Autodesk Fusion 360 part; units mm, degrees
(part 3 of 6)
  spline S34 degree 5 poles (141.8254, 60.2278) (141.8393, 60.255) (141.8664, 60.3097) (141.905, 60.3928) (141.9525, 60.5053) (142.0063, 60.6483) (142.0562, 60.7931) (142.1036, 60.939) (142.1498, 61.0854) (142.1951, 61.2323) (142.2394, 61.3795) (142.2825, 61.5272) (142.3239, 61.6756) (142.3633, 61.8248) (142.4009, 61.9748) (142.4366, 62.1255) (142.4708, 62.2767) (142.5037, 62.4284) (142.5355, 62.5806) (142.5662, 62.7331) (142.5959, 62.886) (142.6244, 63.0393) (142.6517, 63.193) (142.6778, 63.3471) (142.7027, 63.5017) (142.7265, 63.6566) (142.7491, 63.8119) (142.7707, 63.9676) (142.7913, 64.1236) (142.8108, 64.2798) (142.8294, 64.4364) (142.847, 64.5933) (142.8637, 64.7505) (142.8793, 64.908) (142.8939, 65.0657) (142.9076, 65.2238) (142.9204, 65.3821) (142.9322, 65.5407) (142.9431, 65.6995) (142.9532, 65.8586) (142.9623, 66.0179) (142.9705, 66.1775) (142.9779, 66.3372) (142.9844, 66.4972) (142.99, 66.6575) (142.9948, 66.8179) (142.9987, 66.9785) (143.0017, 67.1394) (143.004, 67.3004) (143.0054, 67.4617) (143.006, 67.6231) (143.0057, 67.7847) (143.0047, 67.9465) (143.0028, 68.1085) (143.0002, 68.2706) (142.9967, 68.4329) (142.9925, 68.5954) (142.9875, 68.758) (142.9817, 68.9208) (142.9751, 69.0837) (142.9678, 69.2468) (142.9597, 69.41) (142.9508, 69.5733) (142.9412, 69.7368) (142.9308, 69.9005) (142.9197, 70.0642) (142.9078, 70.2281) (142.8952, 70.3921) (142.8819, 70.5563) (142.8678, 70.7205) (142.853, 70.8848) (142.8406, 71.0164) (142.8309, 71.1152) (142.8243, 71.181) (142.821, 71.2139) knots 0 0 0 0 0 0 0.01428571 0.02857143 0.04285714 0.05714286 0.07142857 0.08571429 0.1 0.11428571 0.12857143 0.14285714 0.15714286 0.17142857 0.18571429 0.2 0.21428571 0.22857143 0.24285714 0.25714286 0.27142857 0.28571429 0.3 0.31428571 0.32857143 0.34285714 0.35714286 0.37142857 0.38571429 0.4 0.41428571 0.42857143 0.44285714 0.45714286 0.47142857 0.48571429 0.5 0.51428571 0.52857143 0.54285714 0.55714286 0.57142857 0.58571429 0.6 0.61428571 0.62857143 0.64285714 0.65714286 0.67142857 0.68571429 0.7 0.71428571 0.72857143 0.74285714 0.75714286 0.77142857 0.78571429 0.8 0.81428571 0.82857143 0.84285714 0.85714286 0.87142857 0.88571429 0.9 0.91428571 0.92857143 0.94285714 0.95714286 0.97142857 0.98571429 1 1 1 1 1 1
  arc A71 (142.821, 71.2139) -> (138.855, 72.8567) centre (111, 0) ccw
  spline S35 degree 5 poles (138.855, 72.8567) (138.8294, 72.8358) (138.7782, 72.7939) (138.7015, 72.7309) (138.5997, 72.6466) (138.473, 72.5409) (138.3469, 72.4347) (138.2214, 72.3281) (138.0965, 72.221) (137.9723, 72.1135) (137.8486, 72.0056) (137.7256, 71.8972) (137.6031, 71.7884) (137.4814, 71.6792) (137.3602, 71.5695) (137.2397, 71.4594) (137.1199, 71.3488) (137.0007, 71.2378) (136.8821, 71.1264) (136.7642, 71.0145) (136.647, 70.9021) (136.5305, 70.7894) (136.4147, 70.6762) (136.2996, 70.5625) (136.1851, 70.4484) (136.0714, 70.3338) (135.9584, 70.2188) (135.8461, 70.1034) (135.7345, 69.9875) (135.6237, 69.8711) (135.5136, 69.7543) (135.4043, 69.637) (135.2957, 69.5193) (135.1879, 69.4011) (135.081, 69.2825) (134.9748, 69.1634) (134.8694, 69.0438) (134.7648, 68.9238) (134.661, 68.8033) (134.5581, 68.6823) (134.456, 68.5608) (134.3548, 68.4389) (134.2545, 68.3165) (134.1551, 68.1936) (134.0566, 68.0702) (133.959, 67.9464) (133.8624, 67.822) (133.7666, 67.6972) (133.6718, 67.5719) (133.578, 67.446) (133.4853, 67.3197) (133.3936, 67.1928) (133.3031, 67.0653) (133.2137, 66.9373) (133.1255, 66.8088) (133.0383, 66.6797) (132.9522, 66.5501) (132.8671, 66.4201) (132.7831, 66.2895) (132.7003, 66.1584) (132.619, 66.0266) (132.5395, 65.894) (132.4619, 65.7606) (132.3863, 65.6264) (132.3123, 65.4914) (132.2395, 65.356) (132.1677, 65.2202) (132.0968, 65.084) (132.0272, 64.9473) (131.9601, 64.8096) (131.897, 64.6704) (131.851, 64.5573) (131.8195, 64.4713) (131.8, 64.4134) (131.7906, 64.3843) knots -1 -1 -1 -1 -1 -1 -0.98571429 -0.97142857 -0.95714286 -0.94285714 -0.92857143 -0.91428571 -0.9 -0.88571429 -0.87142857 -0.85714286 -0.84285714 -0.82857143 -0.81428571 -0.8 -0.78571429 -0.77142857 -0.75714286 -0.74285714 -0.72857143 -0.71428571 -0.7 -0.68571429 -0.67142857 -0.65714286 -0.64285714 -0.62857143 -0.61428571 -0.6 -0.58571429 -0.57142857 -0.55714286 -0.54285714 -0.52857143 -0.51428571 -0.5 -0.48571429 -0.47142857 -0.45714286 -0.44285714 -0.42857143 -0.41428571 -0.4 -0.38571429 -0.37142857 -0.35714286 -0.34285714 -0.32857143 -0.31428571 -0.3 -0.28571429 -0.27142857 -0.25714286 -0.24285714 -0.22857143 -0.21428571 -0.2 -0.18571429 -0.17142857 -0.15714286 -0.14285714 -0.12857143 -0.11428571 -0.1 -0.08571429 -0.07142857 -0.05714286 -0.04285714 -0.02857143 -0.01428571 0 0 0 0 0 0
  line L35 (131.7906, 64.3843) -> (131.5971, 63.7851)
  arc A72 (129.1364, 62.4789) -> (131.5971, 63.7851) centre (129.6939, 64.3996) ccw
  arc A73 (129.1364, 62.4789) -> (126.5329, 63.1765) centre (111, 0) ccw
  arc A74 (125.0549, 65.538) -> (126.5329, 63.1765) centre (127.0104, 65.1187) ccw
  line L36 (125.0549, 65.538) -> (125.1869, 66.1537)
  spline S36 degree 5 poles (125.1869, 66.1537) (125.1933, 66.1836) (125.2054, 66.2435) (125.2212, 66.3338) (125.2379, 66.4547) (125.2529, 66.6068) (125.2636, 66.7596) (125.2716, 66.9128) (125.2783, 67.0662) (125.284, 67.2197) (125.2887, 67.3734) (125.2921, 67.5272) (125.2937, 67.6813) (125.2932, 67.8356) (125.2907, 67.9902) (125.2862, 68.145) (125.2801, 68.2999) (125.2726, 68.455) (125.2639, 68.6102) (125.2541, 68.7655) (125.2432, 68.9208) (125.231, 69.0763) (125.2177, 69.2318) (125.203, 69.3875) (125.187, 69.5432) (125.1699, 69.699) (125.1515, 69.8549) (125.1321, 70.0108) (125.1116, 70.1668) (125.0901, 70.3228) (125.0675, 70.4789) (125.0439, 70.635) (125.0193, 70.7911) (124.9936, 70.9473) (124.9669, 71.1034) (124.9393, 71.2596) (124.9106, 71.4159) (124.881, 71.5721) (124.8504, 71.7284) (124.8189, 71.8846) (124.7865, 72.0409) (124.7532, 72.1971) (124.7189, 72.3533) (124.6838, 72.5096) (124.6477, 72.6658) (124.6108, 72.822) (124.573, 72.9782) (124.5344, 73.1343) (124.4948, 73.2905) (124.4545, 73.4466) (124.4132, 73.6026) (124.3712, 73.7587) (124.3283, 73.9147) (124.2846, 74.0707) (124.2401, 74.2266) (124.1947, 74.3825) (124.1486, 74.5383) (124.1017, 74.6941) (124.0539, 74.8498) (124.0054, 75.0055) (123.9561, 75.1611) (123.9061, 75.3167) (123.8552, 75.4722) (123.8036, 75.6276) (123.7512, 75.783) (123.6981, 75.9383) (123.6442, 76.0935) (123.5896, 76.2487) (123.5342, 76.4037) (123.4781, 76.5587) (123.4213, 76.7137) (123.3752, 76.8375) (123.3403, 76.9304) (123.3169, 76.9923) (123.3052, 77.0233) knots 0 0 0 0 0 0 0.01428571 0.02857143 0.04285714 0.05714286 0.07142857 0.08571429 0.1 0.11428571 0.12857143 0.14285714 0.15714286 0.17142857 0.18571429 0.2 0.21428571 0.22857143 0.24285714 0.25714286 0.27142857 0.28571429 0.3 0.31428571 0.32857143 0.34285714 0.35714286 0.37142857 0.38571429 0.4 0.41428571 0.42857143 0.44285714 0.45714286 0.47142857 0.48571429 0.5 0.51428571 0.52857143 0.54285714 0.55714286 0.57142857 0.58571429 0.6 0.61428571 0.62857143 0.64285714 0.65714286 0.67142857 0.68571429 0.7 0.71428571 0.72857143 0.74285714 0.75714286 0.77142857 0.78571429 0.8 0.81428571 0.82857143 0.84285714 0.85714286 0.87142857 0.88571429 0.9 0.91428571 0.92857143 0.94285714 0.95714286 0.97142857 0.98571429 1 1 1 1 1 1
  arc A75 (123.3052, 77.0233) -> (119.0492, 77.5836) centre (111, 0) ccw
  spline S37 degree 5 poles (119.0492, 77.5836) (119.0298, 77.5567) (118.9912, 77.503) (118.9335, 77.4223) (118.8569, 77.3146) (118.7619, 77.1796) (118.6676, 77.0444) (118.574, 76.909) (118.4811, 76.7732) (118.3889, 76.6373) (118.2973, 76.501) (118.2065, 76.3645) (118.1165, 76.2277) (118.0271, 76.0906) (117.9385, 75.9533) (117.8506, 75.8158) (117.7634, 75.678) (117.677, 75.5399) (117.5913, 75.4016) (117.5065, 75.263) (117.4223, 75.1242) (117.339, 74.9851) (117.2564, 74.8457) (117.1746, 74.7061) (117.0936, 74.5663) (117.0134, 74.4262) (116.934, 74.2859) (116.8554, 74.1453) (116.7776, 74.0045) (116.7007, 73.8634) (116.6246, 73.7221) (116.5493, 73.5805) (116.4749, 73.4387) (116.4014, 73.2966) (116.3288, 73.1543) (116.257, 73.0118) (116.1862, 72.869) (116.1162, 72.726) (116.0472, 72.5828) (115.9791, 72.4393) (115.9119, 72.2956) (115.8457, 72.1516) (115.7805, 72.0074) (115.7163, 71.863) (115.6531, 71.7183) (115.5909, 71.5734) (115.5297, 71.4283) (115.4696, 71.2829) (115.4104, 71.1373) (115.3524, 70.9915) (115.2955, 70.8454) (115.2398, 70.6991) (115.1853, 70.5526) (115.1321, 70.4058) (115.0802, 70.2588) (115.0294, 70.1116) (114.9798, 69.9641) (114.9312, 69.8165) (114.8838, 69.6686) (114.8378, 69.5205) (114.7934, 69.3722) (114.751, 69.2235) (114.7106, 69.0746) (114.6722, 68.9254) (114.6356, 68.7759) (114.6004, 68.6262) (114.5662, 68.4764) (114.533, 68.3265) (114.5011, 68.1765) (114.4719, 68.0261) (114.447, 67.8753) (114.4318, 67.7542) (114.4237, 67.663) (114.4199, 67.602) (114.4183, 67.5715) knots -1 -1 -1 -1 -1 -1 -0.98571429 -0.97142857 -0.95714286 -0.94285714 -0.92857143 -0.91428571 -0.9 -0.88571429 -0.87142857 -0.85714286 -0.84285714 -0.82857143 -0.81428571 -0.8 -0.78571429 -0.77142857 -0.75714286 -0.74285714 -0.72857143 -0.71428571 -0.7 -0.68571429 -0.67142857 -0.65714286 -0.64285714 -0.62857143 -0.61428571 -0.6 -0.58571429 -0.57142857 -0.55714286 -0.54285714 -0.52857143 -0.51428571 -0.5 -0.48571429 -0.47142857 -0.45714286 -0.44285714 -0.42857143 -0.41428571 -0.4 -0.38571429 -0.37142857 -0.35714286 -0.34285714 -0.32857143 -0.31428571 -0.3 -0.28571429 -0.27142857 -0.25714286 -0.24285714 -0.22857143 -0.21428571 -0.2 -0.18571429 -0.17142857 -0.15714286 -0.14285714 -0.12857143 -0.11428571 -0.1 -0.08571429 -0.07142857 -0.05714286 -0.04285714 -0.02857143 -0.01428571 0 0 0 0 0 0
  line L37 (114.4183, 67.5715) -> (114.3865, 66.9426)
  arc A76 (112.3477, 65.044) -> (114.3865, 66.9426) centre (112.3891, 67.0436) ccw
  arc A77 (112.3477, 65.044) -> (109.6523, 65.044) centre (111, 0) ccw
  arc A78 (107.6135, 66.9426) -> (109.6523, 65.044) centre (109.6109, 67.0436) ccw
  line L38 (107.6135, 66.9426) -> (107.5817, 67.5715)
  spline S38 degree 5 poles (107.5817, 67.5715) (107.5801, 67.602) (107.5763, 67.663) (107.5682, 67.7542) (107.553, 67.8753) (107.5281, 68.0261) (107.4989, 68.1765) (107.467, 68.3265) (107.4338, 68.4764) (107.3996, 68.6262) (107.3644, 68.7759) (107.3278, 68.9254) (107.2894, 69.0746) (107.249, 69.2235) (107.2066, 69.3722) (107.1622, 69.5205) (107.1162, 69.6686) (107.0688, 69.8165) (107.0202, 69.9641) (106.9706, 70.1116) (106.9198, 70.2588) (106.8679, 70.4058) (106.8147, 70.5526) (106.7602, 70.6991) (106.7045, 70.8454) (106.6476, 70.9915) (106.5896, 71.1373) (106.5304, 71.2829) (106.4703, 71.4283) (106.4091, 71.5734) (106.3469, 71.7183) (106.2837, 71.863) (106.2195, 72.0074) (106.1543, 72.1516) (106.0881, 72.2956) (106.0209, 72.4393) (105.9528, 72.5828) (105.8838, 72.726) (105.8138, 72.869) (105.743, 73.0118) (105.6712, 73.1543) (105.5986, 73.2966) (105.5251, 73.4387) (105.4507, 73.5805) (105.3754, 73.7221) (105.2993, 73.8634) (105.2224, 74.0045) (105.1446, 74.1453) (105.066, 74.2859) (104.9866, 74.4262) (104.9064, 74.5663) (104.8254, 74.7061) (104.7436, 74.8457) (104.661, 74.9851) (104.5777, 75.1242) (104.4935, 75.263) (104.4087, 75.4016) (104.323, 75.5399) (104.2366, 75.678) (104.1494, 75.8158) (104.0615, 75.9533) (103.9729, 76.0906) (103.8835, 76.2277) (103.7935, 76.3645) (103.7027, 76.501) (103.6111, 76.6373) (103.5189, 76.7732) (103.426, 76.909) (103.3324, 77.0444) (103.2381, 77.1796) (103.1431, 77.3146) (103.0665, 77.4223) (103.0088, 77.503) (102.9702, 77.5567) (102.9508, 77.5836) knots 0 0 0 0 0 0 0.01428571 0.02857143 0.04285714 0.05714286 0.07142857 0.08571429 0.1 0.11428571 0.12857143 0.14285714 0.15714286 0.17142857 0.18571429 0.2 0.21428571 0.22857143 0.24285714 0.25714286 0.27142857 0.28571429 0.3 0.31428571 0.32857143 0.34285714 0.35714286 0.37142857 0.38571429 0.4 0.41428571 0.42857143 0.44285714 0.45714286 0.47142857 0.48571429 0.5 0.51428571 0.52857143 0.54285714 0.55714286 0.57142857 0.58571429 0.6 0.61428571 0.62857143 0.64285714 0.65714286 0.67142857 0.68571429 0.7 0.71428571 0.72857143 0.74285714 0.75714286 0.77142857 0.78571429 0.8 0.81428571 0.82857143 0.84285714 0.85714286 0.87142857 0.88571429 0.9 0.91428571 0.92857143 0.94285714 0.95714286 0.97142857 0.98571429 1 1 1 1 1 1
  arc A79 (102.9508, 77.5836) -> (98.6948, 77.0233) centre (111, 0) ccw
  spline S39 degree 5 poles (98.6948, 77.0233) (98.6831, 76.9923) (98.6597, 76.9304) (98.6248, 76.8375) (98.5787, 76.7137) (98.5219, 76.5587) (98.4658, 76.4037) (98.4104, 76.2487) (98.3558, 76.0935) (98.3019, 75.9383) (98.2488, 75.783) (98.1964, 75.6276) (98.1448, 75.4722) (98.0939, 75.3167) (98.0439, 75.1611) (97.9946, 75.0055) (97.9461, 74.8498) (97.8983, 74.6941) (97.8514, 74.5383) (97.8053, 74.3825) (97.7599, 74.2266) (97.7154, 74.0707) (97.6717, 73.9147) (97.6288, 73.7587) (97.5868, 73.6026) (97.5455, 73.4466) (97.5052, 73.2905) (97.4656, 73.1343) (97.427, 72.9782) (97.3892, 72.822) (97.3523, 72.6658) (97.3162, 72.5096) (97.2811, 72.3533) (97.2468, 72.1971) (97.2135, 72.0409) (97.1811, 71.8846) (97.1496, 71.7284) (97.119, 71.5721) (97.0894, 71.4159) (97.0607, 71.2596) (97.0331, 71.1034) (97.0064, 70.9473) (96.9807, 70.7911) (96.9561, 70.635) (96.9325, 70.4789) (96.9099, 70.3228) (96.8884, 70.1668) (96.8679, 70.0108) (96.8485, 69.8549) (96.8301, 69.699) (96.813, 69.5432) (96.797, 69.3875) (96.7823, 69.2318) (96.769, 69.0763) (96.7568, 68.9208) (96.7459, 68.7655) (96.7361, 68.6102) (96.7274, 68.455) (96.7199, 68.2999) (96.7138, 68.145) (96.7093, 67.9902) (96.7068, 67.8356) (96.7063, 67.6813) (96.7079, 67.5272) (96.7113, 67.3734) (96.716, 67.2197) (96.7217, 67.0662) (96.7284, 66.9128) (96.7364, 66.7596) (96.7471, 66.6068) (96.7621, 66.4547) (96.7788, 66.3338) (96.7946, 66.2435) (96.8067, 66.1836) (96.8131, 66.1537) knots -1 -1 -1 -1 -1 -1 -0.98571429 -0.97142857 -0.95714286 -0.94285714 -0.92857143 -0.91428571 -0.9 -0.88571429 -0.87142857 -0.85714286 -0.84285714 -0.82857143 -0.81428571 -0.8 -0.78571429 -0.77142857 -0.75714286 -0.74285714 -0.72857143 -0.71428571 -0.7 -0.68571429 -0.67142857 -0.65714286 -0.64285714 -0.62857143 -0.61428571 -0.6 -0.58571429 -0.57142857 -0.55714286 -0.54285714 -0.52857143 -0.51428571 -0.5 -0.48571429 -0.47142857 -0.45714286 -0.44285714 -0.42857143 -0.41428571 -0.4 -0.38571429 -0.37142857 -0.35714286 -0.34285714 -0.32857143 -0.31428571 -0.3 -0.28571429 -0.27142857 -0.25714286 -0.24285714 -0.22857143 -0.21428571 -0.2 -0.18571429 -0.17142857 -0.15714286 -0.14285714 -0.12857143 -0.11428571 -0.1 -0.08571429 -0.07142857 -0.05714286 -0.04285714 -0.02857143 -0.01428571 0 0 0 0 0 0
  line L39 (96.8131, 66.1537) -> (96.9451, 65.538)
  arc A80 (95.4671, 63.1765) -> (96.9451, 65.538) centre (94.9896, 65.1187) ccw
  arc A81 (95.4671, 63.1765) -> (92.8636, 62.4789) centre (111, 0) ccw
  arc A82 (90.4029, 63.7851) -> (92.8636, 62.4789) centre (92.3061, 64.3996) ccw
  line L40 (90.4029, 63.7851) -> (90.2094, 64.3843)
  spline S40 degree 5 poles (90.2094, 64.3843) (90.2, 64.4134) (90.1805, 64.4713) (90.149, 64.5573) (90.103, 64.6704) (90.0399, 64.8096) (89.9728, 64.9473) (89.9032, 65.084) (89.8323, 65.2202) (89.7605, 65.356) (89.6877, 65.4914) (89.6137, 65.6264) (89.5381, 65.7606) (89.4605, 65.894) (89.381, 66.0266) (89.2997, 66.1584) (89.2169, 66.2895) (89.1329, 66.4201) (89.0478, 66.5501) (88.9617, 66.6797) (88.8745, 66.8088) (88.7863, 66.9373) (88.6969, 67.0653) (88.6064, 67.1928) (88.5147, 67.3197) (88.422, 67.446) (88.3282, 67.5719) (88.2334, 67.6972) (88.1376, 67.822) (88.041, 67.9464) (87.9434, 68.0702) (87.8449, 68.1936) (87.7455, 68.3165) (87.6452, 68.4389) (87.544, 68.5608) (87.4419, 68.6823) (87.339, 68.8033) (87.2352, 68.9238) (87.1306, 69.0438) (87.0252, 69.1634) (86.919, 69.2825) (86.8121, 69.4011) (86.7043, 69.5193) (86.5957, 69.637) (86.4864, 69.7543) (86.3763, 69.8711) (86.2655, 69.9875) (86.1539, 70.1034) (86.0416, 70.2188) (85.9286, 70.3338) (85.8149, 70.4484) (85.7004, 70.5625) (85.5853, 70.6762) (85.4695, 70.7894) (85.353, 70.9021) (85.2358, 71.0145) (85.1179, 71.1264) (84.9993, 71.2378) (84.8801, 71.3488) (84.7603, 71.4594) (84.6398, 71.5695) (84.5186, 71.6792) (84.3969, 71.7884) (84.2744, 71.8972) (84.1514, 72.0056) (84.0277, 72.1135) (83.9035, 72.221) (83.7786, 72.3281) (83.6531, 72.4347) (83.527, 72.5409) (83.4003, 72.6466) (83.2985, 72.7309) (83.2218, 72.7939) (83.1706, 72.8358) (83.145, 72.8567) knots 0 0 0 0 0 0 0.01428571 0.02857143 0.04285714 0.05714286 0.07142857 0.08571429 0.1 0.11428571 0.12857143 0.14285714 0.15714286 0.17142857 0.18571429 0.2 0.21428571 0.22857143 0.24285714 0.25714286 0.27142857 0.28571429 0.3 0.31428571 0.32857143 0.34285714 0.35714286 0.37142857 0.38571429 0.4 0.41428571 0.42857143 0.44285714 0.45714286 0.47142857 0.48571429 0.5 0.51428571 0.52857143 0.54285714 0.55714286 0.57142857 0.58571429 0.6 0.61428571 0.62857143 0.64285714 0.65714286 0.67142857 0.68571429 0.7 0.71428571 0.72857143 0.74285714 0.75714286 0.77142857 0.78571429 0.8 0.81428571 0.82857143 0.84285714 0.85714286 0.87142857 0.88571429 0.9 0.91428571 0.92857143 0.94285714 0.95714286 0.97142857 0.98571429 1 1 1 1 1 1
  arc A83 (83.145, 72.8567) -> (79.179, 71.2139) centre (111, 0) ccw
  spline S41 degree 5 poles (79.179, 71.2139) (79.1757, 71.181) (79.1691, 71.1152) (79.1594, 71.0164) (79.147, 70.8848) (79.1322, 70.7205) (79.1181, 70.5563) (79.1048, 70.3921) (79.0922, 70.2281) (79.0803, 70.0642) (79.0692, 69.9005) (79.0588, 69.7368) (79.0492, 69.5733) (79.0403, 69.41) (79.0322, 69.2468) (79.0249, 69.0837) (79.0183, 68.9208) (79.0125, 68.758) (79.0075, 68.5954) (79.0033, 68.4329) (78.9998, 68.2706) (78.9972, 68.1085) (78.9953, 67.9465) (78.9943, 67.7847) (78.994, 67.6231) (78.9946, 67.4617) (78.996, 67.3004) (78.9983, 67.1394) (79.0013, 66.9785) (79.0052, 66.8179) (79.01, 66.6575) (79.0156, 66.4972) (79.0221, 66.3372) (79.0295, 66.1775) (79.0377, 66.0179) (79.0468, 65.8586) (79.0569, 65.6995) (79.0678, 65.5407) (79.0796, 65.3821) (79.0924, 65.2238) (79.1061, 65.0657) (79.1207, 64.908) (79.1363, 64.7505) (79.153, 64.5933) (79.1706, 64.4364) (79.1892, 64.2798) (79.2087, 64.1236) (79.2293, 63.9676) (79.2509, 63.8119) (79.2735, 63.6566) (79.2973, 63.5017) (79.3222, 63.3471) (79.3483, 63.193) (79.3756, 63.0393) (79.4041, 62.886) (79.4338, 62.7331) (79.4645, 62.5806) (79.4963, 62.4284) (79.5292, 62.2767) (79.5634, 62.1255) (79.5991, 61.9748) (79.6367, 61.8248) (79.6761, 61.6756) (79.7175, 61.5272) (79.7606, 61.3795) (79.8049, 61.2323) (79.8502, 61.0854) (79.8964, 60.939) (79.9438, 60.7931) (79.9937, 60.6483) (80.0475, 60.5053) (80.095, 60.3928) (80.1336, 60.3097) (80.1607, 60.255) (80.1746, 60.2278) knots -1 -1 -1 -1 -1 -1 -0.98571429 -0.97142857 -0.95714286 -0.94285714 -0.92857143 -0.91428571 -0.9 -0.88571429 -0.87142857 -0.85714286 -0.84285714 -0.82857143 -0.81428571 -0.8 -0.78571429 -0.77142857 -0.75714286 -0.74285714 -0.72857143 -0.71428571 -0.7 -0.68571429 -0.67142857 -0.65714286 -0.64285714 -0.62857143 -0.61428571 -0.6 -0.58571429 -0.57142857 -0.55714286 -0.54285714 -0.52857143 -0.51428571 -0.5 -0.48571429 -0.47142857 -0.45714286 -0.44285714 -0.42857143 -0.41428571 -0.4 -0.38571429 -0.37142857 -0.35714286 -0.34285714 -0.32857143 -0.31428571 -0.3 -0.28571429 -0.27142857 -0.25714286 -0.24285714 -0.22857143 -0.21428571 -0.2 -0.18571429 -0.17142857 -0.15714286 -0.14285714 -0.12857143 -0.11428571 -0.1 -0.08571429 -0.07142857 -0.05714286 -0.04285714 -0.02857143 -0.01428571 0 0 0 0 0 0
  line L41 (80.1746, 60.2278) -> (80.4615, 59.6672)
  arc A84 (79.6451, 57.0036) -> (80.4615, 59.6672) centre (78.6812, 58.756) ccw
  arc A85 (79.6451, 57.0036) -> (77.3109, 55.656) centre (111, 0) ccw
  arc A86 (74.5959, 56.2807) -> (77.3109, 55.656) centre (76.2752, 57.3669) ccw
  line L42 (74.5959, 56.2807) -> (74.2539, 56.8094)
  spline S42 degree 5 poles (74.2539, 56.8094) (74.2373, 56.8351) (74.2035, 56.886) (74.1509, 56.9609) (74.0771, 57.0583) (73.9802, 57.1764) (73.8797, 57.292) (73.7771, 57.406) (73.6734, 57.5192) (73.5688, 57.6318) (73.4635, 57.7438) (73.3571, 57.855) (73.2493, 57.9651) (73.1398, 58.0739) (73.0287, 58.1813) (72.9161, 58.2876) (72.8022, 58.3929) (72.6872, 58.4972) (72.5714, 58.6008) (72.4546, 58.7037) (72.3371, 58.8058) (72.2186, 58.9072) (72.0991, 59.0077) (71.9787, 59.1074) (71.8573, 59.2062) (71.735, 59.3042) (71.6118, 59.4015) (71.4878, 59.498) (71.363, 59.5938) (71.2375, 59.6889) (71.1111, 59.7833) (70.9841, 59.877) (70.8563, 59.97) (70.7277, 60.0623) (70.5984, 60.1538) (70.4684, 60.2447) (70.3376, 60.3349) (70.2062, 60.4245) (70.0741, 60.5133) (69.9414, 60.6015) (69.808, 60.6891) (69.6739, 60.776) (69.5392, 60.8623) (69.4039, 60.9479) (69.2679, 61.0329) (69.1314, 61.1172) (68.9942, 61.2009) (68.8565, 61.284) (68.7181, 61.3665) (68.5792, 61.4483) (68.4397, 61.5295) (68.2996, 61.6101) (68.159, 61.6901) (68.0178, 61.7695) (67.876, 61.8483) (67.7338, 61.9264) (67.5909, 62.004) (67.4476, 62.081) (67.3037, 62.1573) (67.1593, 62.2331) (67.0144, 62.3083) (66.869, 62.3829) (66.7231, 62.4569) (66.5767, 62.5303) (66.4298, 62.6031) (66.2824, 62.6754) (66.1346, 62.747) (65.9862, 62.8181) (65.8374, 62.8886) (65.6882, 62.9586) (65.5384, 63.0279) (65.4183, 63.0829) (65.3279, 63.124) (65.2676, 63.1512) (65.2374, 63.1648) knots 0 0 0 0 0 0 0.01428571 0.02857143 0.04285714 0.05714286 0.07142857 0.08571429 0.1 0.11428571 0.12857143 0.14285714 0.15714286 0.17142857 0.18571429 0.2 0.21428571 0.22857143 0.24285714 0.25714286 0.27142857 0.28571429 0.3 0.31428571 0.32857143 0.34285714 0.35714286 0.37142857 0.38571429 0.4 0.41428571 0.42857143 0.44285714 0.45714286 0.47142857 0.48571429 0.5 0.51428571 0.52857143 0.54285714 0.55714286 0.57142857 0.58571429 0.6 0.61428571 0.62857143 0.64285714 0.65714286 0.67142857 0.68571429 0.7 0.71428571 0.72857143 0.74285714 0.75714286 0.77142857 0.78571429 0.8 0.81428571 0.82857143 0.84285714 0.85714286 0.87142857 0.88571429 0.9 0.91428571 0.92857143 0.94285714 0.95714286 0.97142857 0.98571429 1 1 1 1 1 1
  arc A87 (65.2374, 63.1648) -> (61.8318, 60.5515) centre (111, 0) ccw
  spline S43 degree 5 poles (61.8318, 60.5515) (61.8371, 60.5188) (61.8477, 60.4535) (61.864, 60.3557) (61.886, 60.2253) (61.9143, 60.0628) (61.9432, 59.9005) (61.9728, 59.7385) (62.003, 59.5768) (62.034, 59.4154) (62.0656, 59.2544) (62.098, 59.0936) (62.131, 58.9332) (62.1647, 58.7731) (62.1991, 58.6134) (62.2342, 58.4539) (62.27, 58.2949) (62.3066, 58.1361) (62.3438, 57.9778) (62.3818, 57.8197) (62.4205, 57.6621) (62.4599, 57.5048) (62.5, 57.3478) (62.5409, 57.1913) (62.5825, 57.0351) (62.6248, 56.8794) (62.6679, 56.724) (62.7117, 56.569) (62.7563, 56.4144) (62.8017, 56.2603) (62.8478, 56.1065) (62.8947, 55.9532) (62.9424, 55.8004) (62.9909, 55.6479) (63.0401, 55.496) (63.0902, 55.3444) (63.141, 55.1934) (63.1927, 55.0428) (63.2451, 54.8927) (63.2984, 54.743) (63.3526, 54.5939) (63.4076, 54.4453) (63.4634, 54.2972) (63.5201, 54.1497) (63.5778, 54.0027) (63.6362, 53.8563) (63.6956, 53.7104) (63.7558, 53.5651) (63.817, 53.4203) (63.879, 53.2762) (63.9421, 53.1326) (64.0061, 52.9898) (64.0712, 52.8477) (64.1374, 52.7063) (64.2046, 52.5656) (64.2729, 52.4256) (64.342, 52.2862) (64.4121, 52.1475) (64.4831, 52.0094) (64.5553, 51.8722) (64.6288, 51.7359) (64.7039, 51.6008) (64.7806, 51.4669) (64.859, 51.3342) (64.9389, 51.2027) (65.0198, 51.072) (65.1015, 50.9418) (65.184, 50.8123) (65.2676, 50.6837) (65.3533, 50.5567) (65.4423, 50.4325) (65.5172, 50.3361) (65.576, 50.2659) (65.6164, 50.2201) (65.6369, 50.1974) knots -1 -1 -1 -1 -1 -1 -0.98571429 -0.97142857 -0.95714286 -0.94285714 -0.92857143 -0.91428571 -0.9 -0.88571429 -0.87142857 -0.85714286 -0.84285714 -0.82857143 -0.81428571 -0.8 -0.78571429 -0.77142857 -0.75714286 -0.74285714 -0.72857143 -0.71428571 -0.7 -0.68571429 -0.67142857 -0.65714286 -0.64285714 -0.62857143 -0.61428571 -0.6 -0.58571429 -0.57142857 -0.55714286 -0.54285714 -0.52857143 -0.51428571 -0.5 -0.48571429 -0.47142857 -0.45714286 -0.44285714 -0.42857143 -0.41428571 -0.4 -0.38571429 -0.37142857 -0.35714286 -0.34285714 -0.32857143 -0.31428571 -0.3 -0.28571429 -0.27142857 -0.25714286 -0.24285714 -0.22857143 -0.21428571 -0.2 -0.18571429 -0.17142857 -0.15714286 -0.14285714 -0.12857143 -0.11428571 -0.1 -0.08571429 -0.07142857 -0.05714286 -0.04285714 -0.02857143 -0.01428571 0 0 0 0 0 0
  line L43 (65.6369, 50.1974) -> (66.0591, 49.7302)
  arc A88 (65.9599, 46.946) -> (66.0591, 49.7302) centre (64.5752, 48.3892) ccw
  arc A89 (65.9599, 46.946) -> (64.054, 45.0401) centre (111, 0) ccw
  arc A90 (61.2698, 44.9409) -> (64.054, 45.0401) centre (62.6108, 46.4248) ccw
  line L44 (61.2698, 44.9409) -> (60.8026, 45.3631)
  spline S44 degree 5 poles (60.8026, 45.3631) (60.7799, 45.3836) (60.7341, 45.424) (60.6639, 45.4828) (60.5675, 45.5577) (60.4433, 45.6467) (60.3163, 45.7324) (60.1877, 45.816) (60.0582, 45.8985) (59.928, 45.9802) (59.7973, 46.0611) (59.6658, 46.141) (59.5331, 46.2194) (59.3992, 46.2961) (59.2641, 46.3712) (59.1278, 46.4447) (58.9906, 46.5169) (58.8525, 46.5879) (58.7138, 46.658) (58.5744, 46.7271) (58.4344, 46.7954) (58.2937, 46.8626) (58.1523, 46.9288) (58.0102, 46.9939) (57.8674, 47.0579) (57.7238, 47.121) (57.5797, 47.183) (57.4349, 47.2442) (57.2896, 47.3044) (57.1437, 47.3638) (56.9973, 47.4222) (56.8503, 47.4799) (56.7028, 47.5366) (56.5547, 47.5924) (56.4061, 47.6474) (56.257, 47.7016) (56.1073, 47.7549) (55.9572, 47.8073) (55.8066, 47.859) (55.6556, 47.9098) (55.504, 47.9599) (55.3521, 48.0091) (55.1996, 48.0576) (55.0468, 48.1053) (54.8935, 48.1522) (54.7397, 48.1983) (54.5856, 48.2437) (54.431, 48.2883) (54.276, 48.3321) (54.1206, 48.3752) (53.9649, 48.4175) (53.8087, 48.4591) (53.6522, 48.5) (53.4952, 48.5401) (53.3379, 48.5795) (53.1803, 48.6182) (53.0222, 48.6562) (52.8639, 48.6934) (52.7051, 48.73) (52.5461, 48.7658) (52.3866, 48.8009) (52.2269, 48.8353) (52.0668, 48.869) (51.9064, 48.902) (51.7456, 48.9344) (51.5846, 48.966) (51.4232, 48.997) (51.2615, 49.0272) (51.0995, 49.0568) (50.9372, 49.0857) (50.7747, 49.114) (50.6443, 49.136) (50.5465, 49.1523) (50.4812, 49.1629) (50.4485, 49.1682) knots 0 0 0 0 0 0 0.01428571 0.02857143 0.04285714 0.05714286 0.07142857 0.08571429 0.1 0.11428571 0.12857143 0.14285714 0.15714286 0.17142857 0.18571429 0.2 0.21428571 0.22857143 0.24285714 0.25714286 0.27142857 0.28571429 0.3 0.31428571 0.32857143 0.34285714 0.35714286 0.37142857 0.38571429 0.4 0.41428571 0.42857143 0.44285714 0.45714286 0.47142857 0.48571429 0.5 0.51428571 0.52857143 0.54285714 0.55714286 0.57142857 0.58571429 0.6 0.61428571 0.62857143 0.64285714 0.65714286 0.67142857 0.68571429 0.7 0.71428571 0.72857143 0.74285714 0.75714286 0.77142857 0.78571429 0.8 0.81428571 0.82857143 0.84285714 0.85714286 0.87142857 0.88571429 0.9 0.91428571 0.92857143 0.94285714 0.95714286 0.97142857 0.98571429 1 1 1 1 1 1
  arc A91 (50.4485, 49.1682) -> (47.8352, 45.7626) centre (111, 0) ccw
  spline S45 degree 5 poles (47.8352, 45.7626) (47.8488, 45.7324) (47.876, 45.6721) (47.9171, 45.5817) (47.9721, 45.4616) (48.0414, 45.3118) (48.1114, 45.1626) (48.1819, 45.0138) (48.253, 44.8654) (48.3246, 44.7176) (48.3969, 44.5702) (48.4697, 44.4233) (48.5431, 44.2769) (48.6171, 44.131) (48.6917, 43.9856) (48.7669, 43.8407) (48.8427, 43.6963) (48.919, 43.5524) (48.996, 43.4091) (49.0736, 43.2662) (49.1517, 43.124) (49.2305, 42.9822) (49.3099, 42.841) (49.3899, 42.7004) (49.4705, 42.5603) (49.5517, 42.4208) (49.6335, 42.2819) (49.716, 42.1435) (49.7991, 42.0058) (49.8828, 41.8686) (49.9671, 41.7321) (50.0521, 41.5961) (50.1377, 41.4608) (50.224, 41.3261) (50.3109, 41.192) (50.3985, 41.0586) (50.4867, 40.9259) (50.5755, 40.7938) (50.6651, 40.6624) (50.7553, 40.5316) (50.8462, 40.4016) (50.9377, 40.2723) (51.03, 40.1437) (51.123, 40.0159) (51.2167, 39.8889) (51.3111, 39.7625) (51.4062, 39.637) (51.502, 39.5122) (51.5985, 39.3882) (51.6958, 39.265) (51.7938, 39.1427) (51.8926, 39.0213) (51.9923, 38.9009) (52.0928, 38.7814) (52.1942, 38.6629) (52.2963, 38.5454) (52.3992, 38.4286) (52.5028, 38.3128) (52.6071, 38.1978) (52.7124, 38.0839) (52.8187, 37.9713) (52.9261, 37.8602) (53.0349, 37.7507) (53.145, 37.6429) (53.2562, 37.5365) (53.3682, 37.4312) (53.4808, 37.3266) (53.594, 37.2229) (53.708, 37.1203) (53.8236, 37.0198) (53.9417, 36.9229) (54.0391, 36.8491) (54.114, 36.7965) (54.1649, 36.7627) (54.1906, 36.7461) knots -1 -1 -1 -1 -1 -1 -0.98571429 -0.97142857 -0.95714286 -0.94285714 -0.92857143 -0.91428571 -0.9 -0.88571429 -0.87142857 -0.85714286 -0.84285714 -0.82857143 -0.81428571 -0.8 -0.78571429 -0.77142857 -0.75714286 -0.74285714 -0.72857143 -0.71428571 -0.7 -0.68571429 -0.67142857 -0.65714286 -0.64285714 -0.62857143 -0.61428571 -0.6 -0.58571429 -0.57142857 -0.55714286 -0.54285714 -0.52857143 -0.51428571 -0.5 -0.48571429 -0.47142857 -0.45714286 -0.44285714 -0.42857143 -0.41428571 -0.4 -0.38571429 -0.37142857 -0.35714286 -0.34285714 -0.32857143 -0.31428571 -0.3 -0.28571429 -0.27142857 -0.25714286 -0.24285714 -0.22857143 -0.21428571 -0.2 -0.18571429 -0.17142857 -0.15714286 -0.14285714 -0.12857143 -0.11428571 -0.1 -0.08571429 -0.07142857 -0.05714286 -0.04285714 -0.02857143 -0.01428571 0 0 0 0 0 0
  line L45 (54.1906, 36.7461) -> (54.7193, 36.4041)
  arc A92 (55.344, 33.6891) -> (54.7193, 36.4041) centre (53.6331, 34.7248) ccw
  arc A93 (55.344, 33.6891) -> (53.9964, 31.3549) centre (111, 0) ccw
  arc A94 (51.3328, 30.5385) -> (53.9964, 31.3549) centre (52.244, 32.3188) ccw
  line L46 (51.3328, 30.5385) -> (50.7722, 30.8254)
  spline S46 degree 5 poles (50.7722, 30.8254) (50.745, 30.8393) (50.6903, 30.8664) (50.6072, 30.905) (50.4947, 30.9525) (50.3517, 31.0063) (50.2069, 31.0562) (50.061, 31.1036) (49.9146, 31.1498) (49.7677, 31.1951) (49.6205, 31.2394) (49.4728, 31.2825) (49.3244, 31.3239) (49.1752, 31.3633) (49.0252, 31.4009) (48.8745, 31.4366) (48.7233, 31.4708) (48.5716, 31.5037) (48.4194, 31.5355) (48.2669, 31.5662) (48.114, 31.5959) (47.9607, 31.6244) (47.807, 31.6517) (47.6529, 31.6778) (47.4983, 31.7027) (47.3434, 31.7265) (47.1881, 31.7491) (47.0324, 31.7707) (46.8764, 31.7913) (46.7202, 31.8108) (46.5636, 31.8294) (46.4067, 31.847) (46.2495, 31.8637) (46.092, 31.8793) (45.9343, 31.8939) (45.7762, 31.9076) (45.6179, 31.9204) (45.4593, 31.9322) (45.3005, 31.9431) (45.1414, 31.9532) (44.9821, 31.9623) (44.8225, 31.9705) (44.6628, 31.9779) (44.5028, 31.9844) (44.3425, 31.99) (44.1821, 31.9948) (44.0215, 31.9987) (43.8606, 32.0017) (43.6996, 32.004) (43.5383, 32.0054) (43.3769, 32.006) (43.2153, 32.0057) (43.0535, 32.0047) (42.8915, 32.0028) (42.7294, 32.0002) (42.5671, 31.9967) (42.4046, 31.9925) (42.242, 31.9875) (42.0792, 31.9817) (41.9163, 31.9751) (41.7532, 31.9678) (41.59, 31.9597) (41.4267, 31.9508) (41.2632, 31.9412) (41.0995, 31.9308) (40.9358, 31.9197) (40.7719, 31.9078) (40.6079, 31.8952) (40.4437, 31.8819) (40.2795, 31.8678) (40.1152, 31.853) (39.9836, 31.8406) (39.8848, 31.8309) (39.819, 31.8243) (39.7861, 31.821) knots 0 0 0 0 0 0 0.01428571 0.02857143 0.04285714 0.05714286 0.07142857 0.08571429 0.1 0.11428571 0.12857143 0.14285714 0.15714286 0.17142857 0.18571429 0.2 0.21428571 0.22857143 0.24285714 0.25714286 0.27142857 0.28571429 0.3 0.31428571 0.32857143 0.34285714 0.35714286 0.37142857 0.38571429 0.4 0.41428571 0.42857143 0.44285714 0.45714286 0.47142857 0.48571429 0.5 0.51428571 0.52857143 0.54285714 0.55714286 0.57142857 0.58571429 0.6 0.61428571 0.62857143 0.64285714 0.65714286 0.67142857 0.68571429 0.7 0.71428571 0.72857143 0.74285714 0.75714286 0.77142857 0.78571429 0.8 0.81428571 0.82857143 0.84285714 0.85714286 0.87142857 0.88571429 0.9 0.91428571 0.92857143 0.94285714 0.95714286 0.97142857 0.98571429 1 1 1 1 1 1
  arc A95 (39.7861, 31.821) -> (38.1433, 27.855) centre (111, 0) ccw
  spline S47 degree 5 poles (38.1433, 27.855) (38.1642, 27.8294) (38.2061, 27.7782) (38.2691, 27.7015) (38.3534, 27.5997) (38.4591, 27.473) (38.5653, 27.3469) (38.6719, 27.2214) (38.779, 27.0965) (38.8865, 26.9723) (38.9944, 26.8486) (39.1028, 26.7256) (39.2116, 26.6031) (39.3208, 26.4814) (39.4305, 26.3602) (39.5406, 26.2397) (39.6512, 26.1199) (39.7622, 26.0007) (39.8736, 25.8821) (39.9855, 25.7642) (40.0979, 25.647) (40.2106, 25.5305) (40.3238, 25.4147) (40.4375, 25.2996) (40.5516, 25.1851) (40.6662, 25.0714) (40.7812, 24.9584) (40.8966, 24.8461) (41.0125, 24.7345) (41.1289, 24.6237) (41.2457, 24.5136) (41.363, 24.4043) (41.4807, 24.2957) (41.5989, 24.1879) (41.7175, 24.081) (41.8366, 23.9748) (41.9562, 23.8694) (42.0762, 23.7648) (42.1967, 23.661) (42.3177, 23.5581) (42.4392, 23.456) (42.5611, 23.3548) (42.6835, 23.2545) (42.8064, 23.1551) (42.9298, 23.0566) (43.0536, 22.959) (43.178, 22.8624) (43.3028, 22.7666) (43.4281, 22.6718) (43.554, 22.578) (43.6803, 22.4853) (43.8072, 22.3936) (43.9347, 22.3031) (44.0627, 22.2137) (44.1912, 22.1255) (44.3203, 22.0383) (44.4499, 21.9522) (44.5799, 21.8671) (44.7105, 21.7831) (44.8416, 21.7003) (44.9734, 21.619) (45.106, 21.5395) (45.2394, 21.4619) (45.3736, 21.3863) (45.5086, 21.3123) (45.644, 21.2395) (45.7798, 21.1677) (45.916, 21.0968) (46.0527, 21.0272) (46.1904, 20.9601) (46.3296, 20.897) (46.4427, 20.851) (46.5287, 20.8195) (46.5866, 20.8) (46.6157, 20.7906) knots -1 -1 -1 -1 -1 -1 -0.98571429 -0.97142857 -0.95714286 -0.94285714 -0.92857143 -0.91428571 -0.9 -0.88571429 -0.87142857 -0.85714286 -0.84285714 -0.82857143 -0.81428571 -0.8 -0.78571429 -0.77142857 -0.75714286 -0.74285714 -0.72857143 -0.71428571 -0.7 -0.68571429 -0.67142857 -0.65714286 -0.64285714 -0.62857143 -0.61428571 -0.6 -0.58571429 -0.57142857 -0.55714286 -0.54285714 -0.52857143 -0.51428571 -0.5 -0.48571429 -0.47142857 -0.45714286 -0.44285714 -0.42857143 -0.41428571 -0.4 -0.38571429 -0.37142857 -0.35714286 -0.34285714 -0.32857143 -0.31428571 -0.3 -0.28571429 -0.27142857 -0.25714286 -0.24285714 -0.22857143 -0.21428571 -0.2 -0.18571429 -0.17142857 -0.15714286 -0.14285714 -0.12857143 -0.11428571 -0.1 -0.08571429 -0.07142857 -0.05714286 -0.04285714 -0.02857143 -0.01428571 0 0 0 0 0 0
  line L47 (46.6157, 20.7906) -> (47.2149, 20.5971)
  arc A96 (48.5211, 18.1364) -> (47.2149, 20.5971) centre (46.6004, 18.6939) ccw
  arc A97 (48.5211, 18.1364) -> (47.8235, 15.5329) centre (111, 0) ccw
  arc A98 (45.462, 14.0549) -> (47.8235, 15.5329) centre (45.8813, 16.0104) ccw
  line L48 (45.462, 14.0549) -> (44.8463, 14.1869)
  spline S48 degree 5 poles (44.8463, 14.1869) (44.8164, 14.1933) (44.7565, 14.2054) (44.6662, 14.2212) (44.5453, 14.2379) (44.3932, 14.2529) (44.2404, 14.2636) (44.0872, 14.2716) (43.9338, 14.2783) (43.7803, 14.284) (43.6266, 14.2887) (43.4728, 14.2921) (43.3187, 14.2937) (43.1644, 14.2932) (43.0098, 14.2907) (42.855, 14.2862) (42.7001, 14.2801) (42.545, 14.2726) (42.3898, 14.2639) (42.2345, 14.2541) (42.0792, 14.2432) (41.9237, 14.231) (41.7682, 14.2177) (41.6125, 14.203) (41.4568, 14.187) (41.301, 14.1699) (41.1451, 14.1515) (40.9892, 14.1321) (40.8332, 14.1116) (40.6772, 14.0901) (40.5211, 14.0675) (40.365, 14.0439) (40.2089, 14.0193) (40.0527, 13.9936) (39.8966, 13.9669) (39.7404, 13.9393) (39.5841, 13.9106) (39.4279, 13.881) (39.2716, 13.8504) (39.1154, 13.8189) (38.9591, 13.7865) (38.8029, 13.7532) (38.6467, 13.7189) (38.4904, 13.6838) (38.3342, 13.6477) (38.178, 13.6108) (38.0218, 13.573) (37.8657, 13.5344) (37.7095, 13.4948) (37.5534, 13.4545) (37.3974, 13.4132) (37.2413, 13.3712) (37.0853, 13.3283) (36.9293, 13.2846) (36.7734, 13.2401) (36.6175, 13.1947) (36.4617, 13.1486) (36.3059, 13.1017) (36.1502, 13.0539) (35.9945, 13.0054) (35.8389, 12.9561) (35.6833, 12.9061) (35.5278, 12.8552) (35.3724, 12.8036) (35.217, 12.7512) (35.0617, 12.6981) (34.9065, 12.6442) (34.7513, 12.5896) (34.5963, 12.5342) (34.4413, 12.4781) (34.2863, 12.4213) (34.1625, 12.3752) (34.0696, 12.3403) (34.0077, 12.3169) (33.9767, 12.3052) knots 0 0 0 0 0 0 0.01428571 0.02857143 0.04285714 0.05714286 0.07142857 0.08571429 0.1 0.11428571 0.12857143 0.14285714 0.15714286 0.17142857 0.18571429 0.2 0.21428571 0.22857143 0.24285714 0.25714286 0.27142857 0.28571429 0.3 0.31428571 0.32857143 0.34285714 0.35714286 0.37142857 0.38571429 0.4 0.41428571 0.42857143 0.44285714 0.45714286 0.47142857 0.48571429 0.5 0.51428571 0.52857143 0.54285714 0.55714286 0.57142857 0.58571429 0.6 0.61428571 0.62857143 0.64285714 0.65714286 0.67142857 0.68571429 0.7 0.71428571 0.72857143 0.74285714 0.75714286 0.77142857 0.78571429 0.8 0.81428571 0.82857143 0.84285714 0.85714286 0.87142857 0.88571429 0.9 0.91428571 0.92857143 0.94285714 0.95714286 0.97142857 0.98571429 1 1 1 1 1 1
  arc A99 (33.9767, 12.3052) -> (33.4164, 8.0492) centre (111, 0) ccw
  spline S49 degree 5 poles (33.4164, 8.0492) (33.4433, 8.0298) (33.497, 7.9912) (33.5777, 7.9335) (33.6854, 7.8569) (33.8204, 7.7619) (33.9556, 7.6676) (34.091, 7.574) (34.2268, 7.4811) (34.3627, 7.3889) (34.499, 7.2973) (34.6355, 7.2065) (34.7723, 7.1165) (34.9094, 7.0271) (35.0467, 6.9385) (35.1842, 6.8506) (35.322, 6.7634) (35.4601, 6.677) (35.5984, 6.5913) (35.737, 6.5065) (35.8758, 6.4223) (36.0149, 6.339) (36.1543, 6.2564) (36.2939, 6.1746) (36.4337, 6.0936) (36.5738, 6.0134) (36.7141, 5.934) (36.8547, 5.8554) (36.9955, 5.7776) (37.1366, 5.7007) (37.2779, 5.6246) (37.4195, 5.5493) (37.5613, 5.4749) (37.7034, 5.4014) (37.8457, 5.3288) (37.9882, 5.257) (38.131, 5.1862) (38.274, 5.1162) (38.4172, 5.0472) (38.5607, 4.9791) (38.7044, 4.9119) (38.8484, 4.8457) (38.9926, 4.7805) (39.137, 4.7163) (39.2817, 4.6531) (39.4266, 4.5909) (39.5717, 4.5297) (39.7171, 4.4696) (39.8627, 4.4104) (40.0085, 4.3524) (40.1546, 4.2955) (40.3009, 4.2398) (40.4474, 4.1853) (40.5942, 4.1321) (40.7412, 4.0802) (40.8884, 4.0294) (41.0359, 3.9798) (41.1835, 3.9312) (41.3314, 3.8838) (41.4795, 3.8378) (41.6278, 3.7934) (41.7765, 3.751) (41.9254, 3.7106) (42.0746, 3.6722) (42.2241, 3.6356) (42.3738, 3.6004) (42.5236, 3.5662) (42.6735, 3.533) (42.8235, 3.5011) (42.9739, 3.4719) (43.1247, 3.447) (43.2458, 3.4318) (43.337, 3.4237) (43.398, 3.4199) (43.4285, 3.4183) knots -1 -1 -1 -1 -1 -1 -0.98571429 -0.97142857 -0.95714286 -0.94285714 -0.92857143 -0.91428571 -0.9 -0.88571429 -0.87142857 -0.85714286 -0.84285714 -0.82857143 -0.81428571 -0.8 -0.78571429 -0.77142857 -0.75714286 -0.74285714 -0.72857143 -0.71428571 -0.7 -0.68571429 -0.67142857 -0.65714286 -0.64285714 -0.62857143 -0.61428571 -0.6 -0.58571429 -0.57142857 -0.55714286 -0.54285714 -0.52857143 -0.51428571 -0.5 -0.48571429 -0.47142857 -0.45714286 -0.44285714 -0.42857143 -0.41428571 -0.4 -0.38571429 -0.37142857 -0.35714286 -0.34285714 -0.32857143 -0.31428571 -0.3 -0.28571429 -0.27142857 -0.25714286 -0.24285714 -0.22857143 -0.21428571 -0.2 -0.18571429 -0.17142857 -0.15714286 -0.14285714 -0.12857143 -0.11428571 -0.1 -0.08571429 -0.07142857 -0.05714286 -0.04285714 -0.02857143 -0.01428571 0 0 0 0 0 0
  line L49 (43.4285, 3.4183) -> (44.0574, 3.3865)
  arc A100 (45.956, 1.3477) -> (44.0574, 3.3865) centre (43.9564, 1.3891) ccw
  arc A101 (45.956, 1.3477) -> (45.956, -1.3477) centre (111, 0) ccw
  arc A102 (44.0574, -3.3865) -> (45.956, -1.3477) centre (43.9564, -1.3891) ccw
  line L50 (44.0574, -3.3865) -> (43.4285, -3.4183)
  spline S50 degree 5 poles (43.4285, -3.4183) (43.398, -3.4199) (43.337, -3.4237) (43.2458, -3.4318) (43.1247, -3.447) (42.9739, -3.4719) (42.8235, -3.5011) (42.6735, -3.533) (42.5236, -3.5662) (42.3738, -3.6004) (42.2241, -3.6356) (42.0746, -3.6722) (41.9254, -3.7106) (41.7765, -3.751) (41.6278, -3.7934) (41.4795, -3.8378) (41.3314, -3.8838) (41.1835, -3.9312) (41.0359, -3.9798) (40.8884, -4.0294) (40.7412, -4.0802) (40.5942, -4.1321) (40.4474, -4.1853) (40.3009, -4.2398) (40.1546, -4.2955) (40.0085, -4.3524) (39.8627, -4.4104) (39.7171, -4.4696) (39.5717, -4.5297) (39.4266, -4.5909) (39.2817, -4.6531) (39.137, -4.7163) (38.9926, -4.7805) (38.8484, -4.8457) (38.7044, -4.9119) (38.5607, -4.9791) (38.4172, -5.0472) (38.274, -5.1162) (38.131, -5.1862) (37.9882, -5.257) (37.8457, -5.3288) (37.7034, -5.4014) (37.5613, -5.4749) (37.4195, -5.5493) (37.2779, -5.6246) (37.1366, -5.7007) (36.9955, -5.7776) (36.8547, -5.8554) (36.7141, -5.934) (36.5738, -6.0134) (36.4337, -6.0936) (36.2939, -6.1746) (36.1543, -6.2564) (36.0149, -6.339) (35.8758, -6.4223) (35.737, -6.5065) (35.5984, -6.5913) (35.4601, -6.677) (35.322, -6.7634) (35.1842, -6.8506) (35.0467, -6.9385) (34.9094, -7.0271) (34.7723, -7.1165) (34.6355, -7.2065) (34.499, -7.2973) (34.3627, -7.3889) (34.2268, -7.4811) (34.091, -7.574) (33.9556, -7.6676) (33.8204, -7.7619) (33.6854, -7.8569) (33.5777, -7.9335) (33.497, -7.9912) (33.4433, -8.0298) (33.4164, -8.0492) knots 0 0 0 0 0 0 0.01428571 0.02857143 0.04285714 0.05714286 0.07142857 0.08571429 0.1 0.11428571 0.12857143 0.14285714 0.15714286 0.17142857 0.18571429 0.2 0.21428571 0.22857143 0.24285714 0.25714286 0.27142857 0.28571429 0.3 0.31428571 0.32857143 0.34285714 0.35714286 0.37142857 0.38571429 0.4 0.41428571 0.42857143 0.44285714 0.45714286 0.47142857 0.48571429 0.5 0.51428571 0.52857143 0.54285714 0.55714286 0.57142857 0.58571429 0.6 0.61428571 0.62857143 0.64285714 0.65714286 0.67142857 0.68571429 0.7 0.71428571 0.72857143 0.74285714 0.75714286 0.77142857 0.78571429 0.8 0.81428571 0.82857143 0.84285714 0.85714286 0.87142857 0.88571429 0.9 0.91428571 0.92857143 0.94285714 0.95714286 0.97142857 0.98571429 1 1 1 1 1 1
  arc A103 (33.4164, -8.0492) -> (33.9767, -12.3052) centre (111, 0) ccw
  spline S51 degree 5 poles (33.9767, -12.3052) (34.0077, -12.3169) (34.0696, -12.3403) (34.1625, -12.3752) (34.2863, -12.4213) (34.4413, -12.4781) (34.5963, -12.5342) (34.7513, -12.5896) (34.9065, -12.6442) (35.0617, -12.6981) (35.217, -12.7512) (35.3724, -12.8036) (35.5278, -12.8552) (35.6833, -12.9061) (35.8389, -12.9561) (35.9945, -13.0054) (36.1502, -13.0539) (36.3059, -13.1017) (36.4617, -13.1486) (36.6175, -13.1947) (36.7734, -13.2401) (36.9293, -13.2846) (37.0853, -13.3283) (37.2413, -13.3712) (37.3974, -13.4132) (37.5534, -13.4545) (37.7095, -13.4948) (37.8657, -13.5344) (38.0218, -13.573) (38.178, -13.6108) (38.3342, -13.6477) (38.4904, -13.6838) (38.6467, -13.7189) (38.8029, -13.7532) (38.9591, -13.7865) (39.1154, -13.8189) (39.2716, -13.8504) (39.4279, -13.881) (39.5841, -13.9106) (39.7404, -13.9393) (39.8966, -13.9669) (40.0527, -13.9936) (40.2089, -14.0193) (40.365, -14.0439) (40.5211, -14.0675) (40.6772, -14.0901) (40.8332, -14.1116) (40.9892, -14.1321) (41.1451, -14.1515) (41.301, -14.1699) (41.4568, -14.187) (41.6125, -14.203) (41.7682, -14.2177) (41.9237, -14.231) (42.0792, -14.2432) (42.2345, -14.2541) (42.3898, -14.2639) (42.545, -14.2726) (42.7001, -14.2801) (42.855, -14.2862) (43.0098, -14.2907) (43.1644, -14.2932) (43.3187, -14.2937) (43.4728, -14.2921) (43.6266, -14.2887) (43.7803, -14.284) (43.9338, -14.2783) (44.0872, -14.2716) (44.2404, -14.2636) (44.3932, -14.2529) (44.5453, -14.2379) (44.6662, -14.2212) (44.7565, -14.2054) (44.8164, -14.1933) (44.8463, -14.1869) knots -1 -1 -1 -1 -1 -1 -0.98571429 -0.97142857 -0.95714286 -0.94285714 -0.92857143 -0.91428571 -0.9 -0.88571429 -0.87142857 -0.85714286 -0.84285714 -0.82857143 -0.81428571 -0.8 -0.78571429 -0.77142857 -0.75714286 -0.74285714 -0.72857143 -0.71428571 -0.7 -0.68571429 -0.67142857 -0.65714286 -0.64285714 -0.62857143 -0.61428571 -0.6 -0.58571429 -0.57142857 -0.55714286 -0.54285714 -0.52857143 -0.51428571 -0.5 -0.48571429 -0.47142857 -0.45714286 -0.44285714 -0.42857143 -0.41428571 -0.4 -0.38571429 -0.37142857 -0.35714286 -0.34285714 -0.32857143 -0.31428571 -0.3 -0.28571429 -0.27142857 -0.25714286 -0.24285714 -0.22857143 -0.21428571 -0.2 -0.18571429 -0.17142857 -0.15714286 -0.14285714 -0.12857143 -0.11428571 -0.1 -0.08571429 -0.07142857 -0.05714286 -0.04285714 -0.02857143 -0.01428571 0 0 0 0 0 0
  line L51 (44.8463, -14.1869) -> (45.462, -14.0549)
  arc A104 (47.8235, -15.5329) -> (45.462, -14.0549) centre (45.8813, -16.0104) ccw
  arc A105 (47.8235, -15.5329) -> (48.5211, -18.1364) centre (111, 0) ccw
  arc A106 (47.2149, -20.5971) -> (48.5211, -18.1364) centre (46.6004, -18.6939) ccw
  line L52 (47.2149, -20.5971) -> (46.6157, -20.7906)
  spline S52 degree 5 poles (46.6157, -20.7906) (46.5866, -20.8) (46.5287, -20.8195) (46.4427, -20.851) (46.3296, -20.897) (46.1904, -20.9601) (46.0527, -21.0272) (45.916, -21.0968) (45.7798, -21.1677) (45.644, -21.2395) (45.5086, -21.3123) (45.3736, -21.3863) (45.2394, -21.4619) (45.106, -21.5395) (44.9734, -21.619) (44.8416, -21.7003) (44.7105, -21.7831) (44.5799, -21.8671) (44.4499, -21.9522) (44.3203, -22.0383) (44.1912, -22.1255) (44.0627, -22.2137) (43.9347, -22.3031) (43.8072, -22.3936) (43.6803, -22.4853) (43.554, -22.578) (43.4281, -22.6718) (43.3028, -22.7666) (43.178, -22.8624) (43.0536, -22.959) (42.9298, -23.0566) (42.8064, -23.1551) (42.6835, -23.2545) (42.5611, -23.3548) (42.4392, -23.456) (42.3177, -23.5581) (42.1967, -23.661) (42.0762, -23.7648) (41.9562, -23.8694) (41.8366, -23.9748) (41.7175, -24.081) (41.5989, -24.1879) (41.4807, -24.2957) (41.363, -24.4043) (41.2457, -24.5136) (41.1289, -24.6237) (41.0125, -24.7345) (40.8966, -24.8461) (40.7812, -24.9584) (40.6662, -25.0714) (40.5516, -25.1851) (40.4375, -25.2996) (40.3238, -25.4147) (40.2106, -25.5305) (40.0979, -25.647) (39.9855, -25.7642) (39.8736, -25.8821) (39.7622, -26.0007) (39.6512, -26.1199) (39.5406, -26.2397) (39.4305, -26.3602) (39.3208, -26.4814) (39.2116, -26.6031) (39.1028, -26.7256) (38.9944, -26.8486) (38.8865, -26.9723) (38.779, -27.0965) (38.6719, -27.2214) (38.5653, -27.3469) (38.4591, -27.473) (38.3534, -27.5997) (38.2691, -27.7015) (38.2061, -27.7782) (38.1642, -27.8294) (38.1433, -27.855) knots 0 0 0 0 0 0 0.01428571 0.02857143 0.04285714 0.05714286 0.07142857 0.08571429 0.1 0.11428571 0.12857143 0.14285714 0.15714286 0.17142857 0.18571429 0.2 0.21428571 0.22857143 0.24285714 0.25714286 0.27142857 0.28571429 0.3 0.31428571 0.32857143 0.34285714 0.35714286 0.37142857 0.38571429 0.4 0.41428571 0.42857143 0.44285714 0.45714286 0.47142857 0.48571429 0.5 0.51428571 0.52857143 0.54285714 0.55714286 0.57142857 0.58571429 0.6 0.61428571 0.62857143 0.64285714 0.65714286 0.67142857 0.68571429 0.7 0.71428571 0.72857143 0.74285714 0.75714286 0.77142857 0.78571429 0.8 0.81428571 0.82857143 0.84285714 0.85714286 0.87142857 0.88571429 0.9 0.91428571 0.92857143 0.94285714 0.95714286 0.97142857 0.98571429 1 1 1 1 1 1
  arc A107 (38.1433, -27.855) -> (39.7861, -31.821) centre (111, 0) ccw
  spline S53 degree 5 poles (39.7861, -31.821) (39.819, -31.8243) (39.8848, -31.8309) (39.9836, -31.8406) (40.1152, -31.853) (40.2795, -31.8678) (40.4437, -31.8819) (40.6079, -31.8952) (40.7719, -31.9078) (40.9358, -31.9197) (41.0995, -31.9308) (41.2632, -31.9412) (41.4267, -31.9508) (41.59, -31.9597) (41.7532, -31.9678) (41.9163, -31.9751) (42.0792, -31.9817) (42.242, -31.9875) (42.4046, -31.9925) (42.5671, -31.9967) (42.7294, -32.0002) (42.8915, -32.0028) (43.0535, -32.0047) (43.2153, -32.0057) (43.3769, -32.006) (43.5383, -32.0054) (43.6996, -32.004) (43.8606, -32.0017) (44.0215, -31.9987) (44.1821, -31.9948) (44.3425, -31.99) (44.5028, -31.9844) (44.6628, -31.9779) (44.8225, -31.9705) (44.9821, -31.9623) (45.1414, -31.9532) (45.3005, -31.9431) (45.4593, -31.9322) (45.6179, -31.9204) (45.7762, -31.9076) (45.9343, -31.8939) (46.092, -31.8793) (46.2495, -31.8637) (46.4067, -31.847) (46.5636, -31.8294) (46.7202, -31.8108) (46.8764, -31.7913) (47.0324, -31.7707) (47.1881, -31.7491) (47.3434, -31.7265) (47.4983, -31.7027) (47.6529, -31.6778) (47.807, -31.6517) (47.9607, -31.6244) (48.114, -31.5959) (48.2669, -31.5662) (48.4194, -31.5355) (48.5716, -31.5037) (48.7233, -31.4708) (48.8745, -31.4366) (49.0252, -31.4009) (49.1752, -31.3633) (49.3244, -31.3239) (49.4728, -31.2825) (49.6205, -31.2394) (49.7677, -31.1951) (49.9146, -31.1498) (50.061, -31.1036) (50.2069, -31.0562) (50.3517, -31.0063) (50.4947, -30.9525) (50.6072, -30.905) (50.6903, -30.8664) (50.745, -30.8393) (50.7722, -30.8254) knots -1 -1 -1 -1 -1 -1 -0.98571429 -0.97142857 -0.95714286 -0.94285714 -0.92857143 -0.91428571 -0.9 -0.88571429 -0.87142857 -0.85714286 -0.84285714 -0.82857143 -0.81428571 -0.8 -0.78571429 -0.77142857 -0.75714286 -0.74285714 -0.72857143 -0.71428571 -0.7 -0.68571429 -0.67142857 -0.65714286 -0.64285714 -0.62857143 -0.61428571 -0.6 -0.58571429 -0.57142857 -0.55714286 -0.54285714 -0.52857143 -0.51428571 -0.5 -0.48571429 -0.47142857 -0.45714286 -0.44285714 -0.42857143 -0.41428571 -0.4 -0.38571429 -0.37142857 -0.35714286 -0.34285714 -0.32857143 -0.31428571 -0.3 -0.28571429 -0.27142857 -0.25714286 -0.24285714 -0.22857143 -0.21428571 -0.2 -0.18571429 -0.17142857 -0.15714286 -0.14285714 -0.12857143 -0.11428571 -0.1 -0.08571429 -0.07142857 -0.05714286 -0.04285714 -0.02857143 -0.01428571 0 0 0 0 0 0
  line L53 (50.7722, -30.8254) -> (51.3328, -30.5385)
  arc A108 (53.9964, -31.3549) -> (51.3328, -30.5385) centre (52.244, -32.3188) ccw
  arc A109 (53.9964, -31.3549) -> (55.344, -33.6891) centre (111, 0) ccw
  arc A110 (54.7193, -36.4041) -> (55.344, -33.6891) centre (53.6331, -34.7248) ccw
  line L54 (54.7193, -36.4041) -> (54.1906, -36.7461)